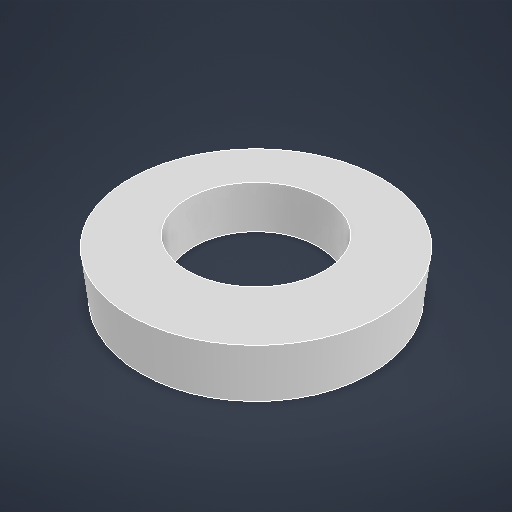
# Autodesk Inventor part: Front_Wheel_Support_2_Test
Saved by Autodesk Inventor 2025 (Build 290162000, 162)
## iProperties
Created: 2024-07-01
Part Number: Front_Wheel_Support_2_Test
Material: Generic
Document SubType Name: Modeling
Designer: Garfieldcmix
Density: 1 g/cm^3
Appearance: Default
Author: Garfieldcmix
Autodesk Inventor part; units mm, degrees
ref_plane "YZ Plane" through (0, 0, 0) normal (1, 0, 0) x (0, 1, 0)
ref_plane "XZ Plane" through (0, 0, 0) normal (0, 1, 0) x (-1, 0, 0)
ref_plane "XY Plane" through (0, 0, 0) normal (0, 0, 1) x (1, 0, 0)
sketch "Sketch1" plane through (0, 0, 0) normal (0, 1, 0) x (-1, 0, 0)
  circle A0 centre (0, 0) radius 2
  circle A1 centre (0, 0) radius 4
  dimension "d0" = 4
  dimension "d1" = 8
  constraints: 2 centre point, 2 coincident
  measures "d0" diameter of A0
  measures "d1" diameter of A1
extrude "Extrusion1" add sketch "Sketch1" along normal blind 1.5
offset faces "Size1" outward -0.18 faces at (-1.9935, 1, -0.1609)
body "Solid1"
